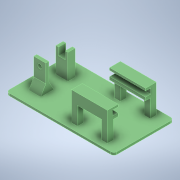
# Autodesk Inventor part: 机架
Saved by Autodesk Inventor 2022 (Build 260153000, 153)
## iProperties
Created: 2022-05-22
Part Number: 机架
Material: 常规
Document SubType Name: Modeling
Designer: zhcne
Density: 1 g/cm^3
Appearance: 平滑 - 深森林绿
Author: zhcne
Autodesk Inventor part; units mm, degrees
ref_plane "YZ Plane" through (0, 0, 0) normal (1, 0, 0) x (0, 1, 0)
ref_plane "XZ Plane" through (0, 0, 0) normal (0, 1, 0) x (-1, 0, 0)
ref_plane "XY Plane" through (0, 0, 0) normal (0, 0, 1) x (1, 0, 0)
sketch "草图1" plane through (0, 0, 0) normal (0, 1, 0) x (-1, 0, 0)
  line L0 (85, -50) -> (-85, -50)
  line L1 (-90, -45) -> (-90, 45)
  line L2 (-85, 50) -> (85, 50)
  line L3 (90, 45) -> (90, -45)
  line L4 (0, 0) -> (0, -30.3694)
  line L5 (0, 0) -> (-59.6627, 0)
  arc A0 (85, -50) -> (90, -45) centre (85, -45) ccw
  arc A1 (90, 45) -> (85, 50) centre (85, 45) ccw
  arc A2 (-85, 50) -> (-90, 45) centre (-85, 45) ccw
  arc A3 (-90, -45) -> (-85, -50) centre (-85, -45) ccw
  point P0 (90, -50)
  point P1 (-90, 50)
  point P2 (-90, -50)
  dimension "d0" = 180
  dimension "d1" = 100
  dimension "d2" = 5
  constraints: 12 end point, 8 point on circle, 8 tangent, 6 point on line, 4 centre point, 3 equal radius, 2 horizontal, 2 parallel, 1 perpendicular, 1 vertical, 2 other
  measures "d0" distance of point (90, -50) point (-90, -50)
  measures "d1" distance of point (-90, -50) point (-90, 50)
  measures "d2" radius of A0
extrude "拉伸1" add sketch "草图1" along normal blind 4
sketch "草图2" plane through (0, 4, 0) normal (0, 1, 0) x (1, 0, 0)
  line L0 (20, 40.9) -> (10, 40.9)
  line L1 (10, 40.9) -> (10, 30.9)
  line L2 (10, 30.9) -> (20, 30.9)
  line L3 (20, 30.9) -> (20, 40.9)
  line L4 (60, 40.9) -> (70, 40.9)
  line L5 (70, 40.9) -> (70, 30.9)
  line L6 (70, 30.9) -> (60, 30.9)
  line L7 (60, 30.9) -> (60, 40.9)
  line L8 (60, -30.9) -> (70, -30.9)
  line L9 (70, -30.9) -> (70, -40.9)
  line L10 (70, -40.9) -> (60, -40.9)
  line L11 (60, -40.9) -> (60, -30.9)
  line L12 (10, -30.9) -> (20, -30.9)
  line L13 (20, -30.9) -> (20, -40.9)
  line L14 (20, -40.9) -> (10, -40.9)
  line L15 (10, -40.9) -> (10, -30.9)
  line L16 (0, 0) -> (216.0528, 0)
  line L17 (0, 0) -> (0, -71.0339)
  dimension "d5" = 61.8
  dimension "d6" = 10
  dimension "d7" = 10
  dimension "d8" = 40
  dimension "d9" = 20
  constraints: 36 end point, 8 parallel, 8 point on line, 5 horizontal, 4 perpendicular, 1 collinear, 1 vertical, 2 other
  measures "d5" distance between parallel lines of L8 L6
  measures "d6" distance of L12.start L12.end
  measures "d7" distance of L12.end L13.end
  measures "d8" distance between parallel lines of L11 L13
  measures "d9" diameter of L15 L17
extrude "拉伸2" add sketch "草图2" along normal blind 30
sketch "草图3" plane through (0, 34, 0) normal (0, 1, 0) x (1, 0, 0)
  line L0 (60, 30.9) -> (70, 30.9) projected
  line L1 (70, 30.9) -> (70, 40.9) projected
  line L2 (70, 30.9) -> (70, 40.9)
  line L3 (10, 40.9) -> (10, 30.9) projected
  line L4 (70, 40.9) -> (10, 40.9)
  line L5 (10, 40.9) -> (10, 30.9)
  line L6 (10, -30.9) -> (10, -40.9)
  line L7 (60, -40.9) -> (70, -40.9) projected
  line L8 (10, -40.9) -> (70, -40.9)
  line L9 (70, -30.9) -> (70, -40.9) projected
  line L10 (70, -40.9) -> (70, -30.9)
  line L11 (70, 40.9) -> (70, 30.9) projected
  line L12 (70, 30.9) -> (70, 22.9)
  line L13 (70, 22.9) -> (10, 22.9)
  line L14 (10, 22.9) -> (10, 30.9)
  line L15 (70, -40.9) -> (70, -30.9) projected
  line L16 (70, -30.9) -> (70, -22.9)
  line L17 (70, -22.9) -> (10, -22.9)
  line L18 (10, -22.9) -> (10, -30.9)
  point P0 (0, 0)
  dimension "d14" = 18
  dimension "d15" = 18
  constraints: 24 end point, 8 perpendicular, 2 vertical, 1 point on line
  measures "d14" distance of L7.end L16.end
  measures "d15" distance of L1.end L12.end
extrude "拉伸3" add sketch "草图3" along normal blind 5
sketch "草图4" plane through (0, 39, 0) normal (0, 1, 0) x (1, 0, 0)
  line L0 (70, 40.9) -> (10, 40.9) projected
  line L1 (10, 40.9) -> (70, 40.9)
  line L2 (70, 40.9) -> (70, 31.9)
  line L3 (70, 22.9) -> (70, 40.9) projected
  line L4 (70, 31.9) -> (10, 31.9)
  line L5 (10, 31.9) -> (10, 40.9)
  line L6 (70, -30.9) -> (70, -40.9) projected
  line L7 (10, -22.9) -> (10, -40.9) projected
  line L8 (70, -40.9) -> (10, -40.9)
  line L9 (10, -40.9) -> (10, -31.9)
  line L10 (10, -31.9) -> (70, -31.9)
  line L11 (70, -31.9) -> (70, -40.9)
  point P0 (0, 0)
  constraints: 16 end point, 3 perpendicular, 2 horizontal, 2 midpoint, 1 collinear, 1 point on line
extrude "拉伸4" add sketch "草图4" along normal blind 9
sketch "草图5" plane through (0, 48, 0) normal (0, 1, 0) x (1, 0, 0)
  line L0 (10, 40.9) -> (20, 40.9) projected
  line L1 (10, 30.9) -> (10, 22.9) projected
  line L2 (10, 40.9) -> (10, 22.9)
  line L3 (70, 22.9) -> (70, 30.9) projected
  line L4 (10, 22.9) -> (70, 22.9)
  line L5 (70, 40.9) -> (70, 30.9) projected
  line L6 (70, 22.9) -> (70, 40.9)
  line L7 (70, 40.9) -> (10, 40.9)
  line L8 (10, -22.9) -> (70, -22.9)
  line L9 (70, -40.9) -> (60, -40.9) projected
  line L10 (70, -22.9) -> (70, -40.9)
  line L11 (20, -40.9) -> (10, -40.9) projected
  line L12 (70, -40.9) -> (10, -40.9)
  line L13 (10, -40.9) -> (10, -22.9)
  point P0 (0, 0)
  constraints: 16 end point, 6 perpendicular, 1 parallel, 1 point on line, 1 vertical
extrude "拉伸5" add sketch "草图5" along normal blind 4
sketch "草图6" plane through (0, 4, 0) normal (0, 1, 0) x (1, 0, 0)
  line L0 (-73, 28) -> (-73, 16)
  line L1 (-73, 16) -> (-53, 16)
  line L2 (-53, 16) -> (-53, 28)
  line L3 (-53, 28) -> (-73, 28)
  line L4 (-90, 45) -> (-90, -45) projected
  line L5 (85, 50) -> (-85, 50) projected
  point P0 (0, 0)
  dimension "d20" = 17
  dimension "d21" = 20
  dimension "d22" = 12
  dimension "d23" = 22
  constraints: 8 end point, 3 perpendicular, 1 vertical
  measures "d20" distance between parallel lines of L4 L0
  measures "d21" distance of L2.end L0.start
  measures "d22" distance of L1.end L2.end
  measures "d23" distance between parallel lines of L5 L3
extrude "拉伸6" add sketch "草图6" along normal blind 29
sketch "草图7" plane through (0, 33, 0) normal (0, 1, 0) x (1, 0, 0)
  line L0 (-53, 28) -> (-53, 16) projected
  line L1 (-53, 28) -> (-53, 16)
  line L2 (-53, 16) -> (-57.5, 16)
  line L3 (-53, 16) -> (-73, 16) projected
  line L4 (-57.5, 16) -> (-57.5, 28)
  line L5 (-53, 28) -> (-73, 28) projected
  line L6 (-57.5, 28) -> (-53, 28)
  line L7 (-73, 16) -> (-73, 28) projected
  line L8 (-73, 28) -> (-73, 16)
  line L9 (-73, 16) -> (-68.5, 16)
  line L10 (-68.5, 16) -> (-68.5, 28)
  line L11 (-73, 28) -> (-68.5, 28)
  point P0 (0, 0)
  dimension "d26" = 4.5
  dimension "d27" = 4.5
  constraints: 16 end point, 4 collinear, 4 point on line, 2 perpendicular
  measures "d26" distance of L0.end L2.end
  measures "d27" distance of L3.end L9.end
extrude "拉伸7" add sketch "草图7" along normal blind 13 contours L0 L2 L4 L5 | L10 L3 L7 L5
sketch "草图8" plane through (0, 4, 0) normal (0, 1, 0) x (1, 0, 0)
  line L0 (-73, -21) -> (-53, -21)
  line L1 (-73, 16) -> (-68.5, 16) projected
  line L2 (-73, -21) -> (-73, -16)
  line L3 (-73, -16) -> (-53, -16)
  line L4 (-53, -16) -> (-53, -21)
  line L5 (-73, 28) -> (-73, 16) projected
  point P0 (0, 0)
  dimension "d30" = 37
  dimension "d31" = 5
  dimension "d32" = 20
  constraints: 8 end point, 2 perpendicular, 1 collinear, 1 horizontal, 1 vertical
  measures "d30" distance between parallel lines of L1 L0
  measures "d31" distance of L0.start L2.end
  measures "d32" distance of L2.end L3.end
extrude "拉伸8" add sketch "草图8" along normal blind 45
sketch "草图9" plane through (-73, 4, 21) normal (0, 0, 1) x (1, 0, 0)
  circle A0 centre (10, 35.099) radius 3.6
  line L0 (20, 45) -> (0, 45) projected
  line L1 (10, 45) -> (10, 16.6489)
  line L2 (-12, 0) -> (158, 0) projected
  point P0 (73, -4)
  dimension "d35" = 7.2
  dimension "d36" = 35.099
  constraints: 2 end point, 1 centre point, 1 midpoint, 1 point on line, 1 vertical
  measures "d35" diameter of A0
  measures "d36" distance from line of L2 A0.centre
extrude "拉伸9" cut sketch "草图9" against normal blind 10
sketch "草图10" plane through (-73, 4, 16) normal (-1, 0, 0) x (0, 0, 1)
  line L0 (0.0194, -1.086) -> (0.0194, 15)
  line L1 (0.0194, 15) -> (-8.9806, -1.086)
  line L2 (-8.9806, -1.086) -> (0.0194, -1.086)
  line L3 (5.1314, -1.086) -> (14.1314, -1.086)
  line L4 (14.1314, -1.086) -> (5, 15)
  line L5 (5, 15) -> (5, 0)
  line L6 (5, 0) -> (13.5149, 0)
  point P0 (-16, -4)
  dimension "d39" = 9
  dimension "d40" = 9
  dimension "d41" = 15
  constraints: 14 end point, 3 point on line, 1 horizontal alignment, 1 perpendicular, 1 vertical
  measures "d39" distance of L3.start L3.end
  measures "d40" distance of L1.end L0.start
  measures "d41" distance of L4.end L5.end
extrude "拉伸11" add sketch "草图10" against normal blind 20
